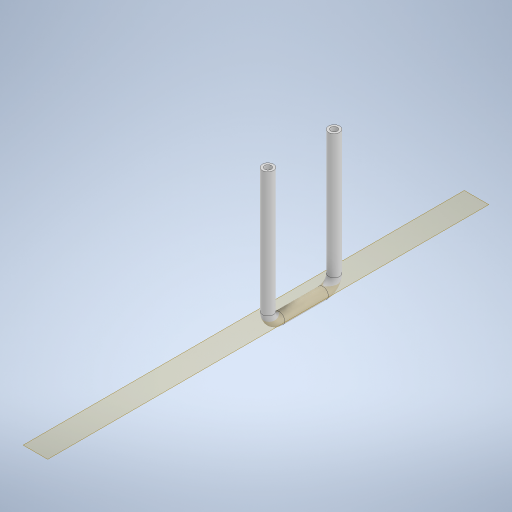
# Autodesk Inventor part: Seat Link
Saved by Autodesk Inventor 2024 (Build 280153000, 153)
## iProperties
Created: 2023-10-22
Part Number: Seat Link
Material: Generic
Document SubType Name: Modeling
Designer: tinas
Density: 1 g/cm^3
Appearance: Default
Author: tinas
Autodesk Inventor part; units mm, degrees
ref_plane "YZ Plane" through (0, 0, 0) normal (1, 0, 0) x (0, 1, 0)
ref_plane "XY Plane" through (0, 0, 0) normal (0, 0, 1) x (1, 0, 0)
sketch "Sketch1" plane through (0, 0, 0) normal (0, 0, 1) x (1, 0, 0)
  circle A0 centre (0, 0) radius 7.5
  circle A1 centre (0, 0) radius 12.5
  dimension "d0" = 15
  dimension "d1" = 25
  constraints: 2 centre point, 2 coincident
  measures "d0" diameter of A0
  measures "d1" diameter of A1
extrude "Extrusion1" add sketch "Sketch1" along normal blind 698
ref_plane "Work Plane2" through (0, 12.5, 0) normal (0, 1, 0) x (-1, 0, 0)
sketch "Sketch3" plane through (0, 12.5, 0) normal (0, 1, 0) x (-1, 0, 0)
  line L0 (219.2482, 398) -> (-262.0284, 398)
  line L1 (12.5, 698) -> (-12.5, 698) projected
  line L2 (351.4203, 300) -> (-288.0764, 300)
  line L3 (12.5, 0) -> (-12.5, 0) projected
  point P0 (0, 0)
  dimension "d7" = 300
  dimension "d8" = 300
  constraints: 4 end point, 2 horizontal
  measures "d7" distance between parallel lines of L0 L1
  measures "d8" distance between parallel lines of L2 L3
bend part "Bend Part1" radius 12.7 angle 90 line through (-219.2482, 12.5, 398) along (1, 0, 0) centre toward (0, 1, 0) moving side (0, 0, 1) both sides no
sketch "Sketch4" plane through (0, 12.5, 0) normal (0, 1, 0) x (-1, 0, 0)
  line L0 (312.7899, 300) -> (-276.8847, 300)
  line L1 (12.5, 0) -> (-12.5, 0) projected
  point P0 (0, 0)
  dimension "d11" = 300
  constraints: 2 end point, 1 horizontal
  measures "d11" distance between parallel lines of L0 L1
bend part "Bend Part2" radius 12.7 angle 90 line through (-312.7899, 12.5, 300) along (1, 0, 0) centre toward (0, 1, 0) moving side (0, 0, -1) both sides no
body "Solid1"
